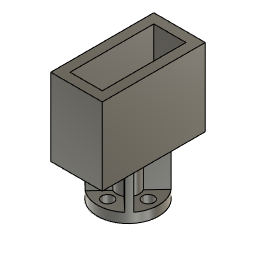
gripper (Autodesk Fusion 360 design; units mm, degrees)
Autodesk Fusion 360 part; units mm, degrees
cylinder "CylinderPrimitive1" add diameter 19 height 3 placed x (1, 0, 0) y (0, 1, 0) z (0, 0, 1) at (0, 0, 0) makes body 1
cylinder "CylinderPrimitive2" add diameter 7 height 11 placed x (1, 0, 0) y (0, 1, 0) z (0, 0, 1) at (0, 0, 3) bodies 1
sketch "Sketch3" plane through (0, 0, 3) normal (0, 0, 1) x (-1, 0, 0)
  circle A0 centre (0, 0) radius 3.5
  circle A1 centre (0, 0) radius 9.5
  circle A2 centre (0, -6.3) radius 1.8
  circle A3 centre (6.3, 0) radius 1.8
  circle A4 centre (0, 6.3) radius 1.8
  circle A5 centre (-6.3, 0) radius 1.8
  line L0 (1.7704, -3.0192) -> (3.1161, -1.5937)
  line L1 (3.1161, -1.5937) -> (7.5441, -5.7738)
  line L2 (6.1984, -7.1993) -> (1.7704, -3.0192)
  arc A6 (6.1984, -7.1993) -> (7.5441, -5.7738) centre (0, 0) ccw
  arc A7 (1.7704, -3.0192) -> (3.1161, -1.5937) centre (0, 0) ccw
  line L3 (7.1993, 6.1984) -> (3.0192, 1.7704)
  arc A8 (3.0192, 1.7704) -> (1.5937, 3.1161) centre (0, 0) ccw
  line L4 (1.5937, 3.1161) -> (5.7738, 7.5441)
  arc A9 (7.1993, 6.1984) -> (5.7738, 7.5441) centre (0, 0) ccw
  line L5 (-6.1984, 7.1993) -> (-1.7704, 3.0192)
  arc A10 (-1.7704, 3.0192) -> (-3.1161, 1.5937) centre (0, 0) ccw
  line L6 (-3.1161, 1.5937) -> (-7.5441, 5.7738)
  arc A11 (-6.1984, 7.1993) -> (-7.5441, 5.7738) centre (0, 0) ccw
  line L7 (-7.1993, -6.1984) -> (-3.0192, -1.7704)
  arc A12 (-3.0192, -1.7704) -> (-1.5937, -3.1161) centre (0, 0) ccw
  line L8 (-1.5937, -3.1161) -> (-5.7738, -7.5441)
  arc A13 (-7.1993, -6.1984) -> (-5.7738, -7.5441) centre (0, 0) ccw
  dimension "d5" = 3.6
  dimension "d6" = 6.3
  dimension "d18" = 360
  dimension "d23" = 360
  constraint perpendicular L0 L1
  constraint parallel L1 L2
  constraint coincident A0 L0.end
  constraint coincident A0 L0.start
  constraint tangent A1 A6
  constraint coincident A1 L1.end
  measures "d5" diameter of A2
  measures "d6" distance of A0.centre A2.centre
sketch "Sketch5" plane through (0, 0, 14) normal (0, 0, 1) x (-1, 0, 0)
  circle A0 centre (0, 0) radius 3.5
  line L0 (8, 16) -> (-8, 16)
  line L1 (-8, 16) -> (-8, -16)
  line L2 (-8, -16) -> (8, -16)
  line L3 (8, -16) -> (8, 16)
  line L4 (8, 16) -> (-8, -16) construction
  line L5 (-8, 16) -> (8, -16) construction
  line L6 (5, 13) -> (-5, 13)
  line L7 (-5, 13) -> (-5, -13)
  line L8 (-5, -13) -> (5, -13)
  line L9 (5, -13) -> (5, 13)
  line L10 (5, 13) -> (-5, -13) construction
  line L11 (-5, 13) -> (5, -13) construction
  dimension "d7" = 16
  dimension "d8" = 32
  dimension "d9" = 10
  dimension "d10" = 26
  constraint horizontal L0
  constraint perpendicular L0 L1
  constraint parallel L0 L2
  constraint parallel L1 L3
  constraint coincident L4 A0.centre
  constraint coincident L5 A0.centre
  constraint coincident A0.centre origin
  constraint horizontal L6
  constraint perpendicular L6 L7
  constraint parallel L6 L8
  constraint parallel L7 L9
  constraint coincident L10 A0.centre
  constraint coincident L11 A0.centre
  measures "d7" distance of L1.end L2.end
  measures "d8" distance of L0.end L1.end
  measures "d9" distance of L7.end L8.end
  measures "d10" distance of L6.end L7.end
extrude "Extrude1" add sketch "Sketch5" along normal blind 24 separate body contours L0 L1 L2 L3 makes body 2
extrude "Extrude2" add sketch "Sketch5" along normal blind 6 contours L6 L7 L8 L9 bodies 1 2
extrude "Extrude3" add sketch "Sketch5" along normal blind 6 contours A0 bodies 1
extrude "Extrude4" cut sketch "Sketch3" against normal blind 4 contours A2 | A3 | A4 | A5 bodies 1
form "Form1" [no effect]
sketch "Sketch9" plane through (0, 0, 0) normal (0, 1, 0) x (1, 0, 0)
extrude "Extrude5" add sketch "Sketch3" along normal blind 11 contours A0 A1 L3 A8 L4 A9 | A0 A1 L1 L2 A6 A7 | A0 A1 L5 A10 L6 A11 | A0 A1 L7 A12 L8 A13 bodies 1
